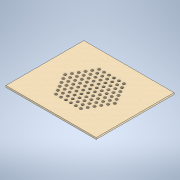
# Autodesk Inventor part: topPlatte
Saved by Autodesk Inventor 2020 (Build 240168000, 168)
## iProperties
Created: 2022-03-26
Part Number: topPlatte
Material: Pappel
Document SubType Name: Modeling
Designer: Eric
Density: 0.448 g/cm^3
Appearance: Pappel
Author: Eric
Autodesk Inventor part; units mm, degrees
ref_plane "YZ Plane" through (0, 0, 0) normal (1, 0, 0) x (0, 1, 0)
ref_plane "XZ Plane" through (0, 0, 0) normal (0, 1, 0) x (-1, 0, 0)
ref_plane "XY Plane" through (0, 0, 0) normal (0, 0, 1) x (1, 0, 0)
sketch "Skizze1" plane through (0, 0, 0) normal (0, 1, 0) x (-1, 0, 0)
  line L0 (0, 0) -> (-218, 0)
  line L1 (-218, 0) -> (-218, 188)
  line L2 (-218, 188) -> (0, 188)
  line L3 (0, 188) -> (0, 0)
  dimension "d0" = 188
  dimension "d1" = 218
  constraints: 8 end point, 2 parallel, 1 horizontal, 1 perpendicular
  measures "d0" distance of L2.end L0.start
  measures "d1" distance of L0.start L0.end
extrude "Extrusion1" add sketch "Skizze1" along normal blind 4
sketch "Skizze2" plane through (0, 0, 0) normal (0, -1, 0) x (1, 0, 0)
  circle A0 centre (109, 94) radius 3
  line L0 (103, 104.3923) -> (115, 104.3923) construction
  line L1 (115, 104.3923) -> (121, 94) construction
  line L2 (121, 94) -> (115, 83.6077) construction
  line L3 (115, 83.6077) -> (103, 83.6077) construction
  line L4 (103, 83.6077) -> (97, 94) construction
  line L5 (97, 94) -> (103, 104.3923) construction
  line L6 (97, 114.7846) -> (121, 114.7846) construction
  line L7 (121, 114.7846) -> (133, 94) construction
  line L8 (133, 94) -> (121, 73.2154) construction
  line L9 (121, 73.2154) -> (97, 73.2154) construction
  line L10 (97, 73.2154) -> (85, 94) construction
  line L11 (85, 94) -> (97, 114.7846) construction
  line L12 (85, 135.5692) -> (133, 135.5692) construction
  line L13 (157, 94) -> (133, 52.4308) construction
  line L14 (133, 52.4308) -> (85, 52.4308) construction
  line L15 (85, 52.4308) -> (61, 94) construction
  line L16 (61, 94) -> (85, 135.5692) construction
  line L17 (0, 0) -> (0, 188) projected
  line L18 (218, 0) -> (0, 0) construction
  line L19 (0, 0) -> (0, 188) projected
  line L20 (0, 94) -> (109, 94) construction
  line L21 (109, 94) -> (109, 0) construction
  line L22 (218, 0) -> (0, 0) construction
  circle A1 centre (103, 104.3923) radius 3
  circle A2 centre (115, 104.3923) radius 3
  circle A3 centre (121, 94) radius 3
  circle A4 centre (115, 83.6077) radius 3
  circle A5 centre (103, 83.6077) radius 3
  circle A6 centre (97, 94) radius 3
  circle A7 centre (85, 94) radius 3
  circle A8 centre (91, 104.3923) radius 3
  circle A9 centre (97, 114.7846) radius 3
  circle A10 centre (121, 114.7846) radius 3
  circle A11 centre (127, 104.3923) radius 3
  circle A12 centre (109, 114.7846) radius 3
  circle A13 centre (133, 94) radius 3
  circle A14 centre (127, 83.6077) radius 3
  circle A15 centre (121, 73.2154) radius 3
  circle A16 centre (109, 73.2154) radius 3
  circle A17 centre (97, 73.2154) radius 3
  circle A18 centre (91, 83.6077) radius 3
  circle A19 centre (85, 135.5692) radius 3
  circle A20 centre (73, 114.7846) radius 3
  circle A21 centre (79, 125.1769) radius 3
  circle A22 centre (67, 104.3923) radius 3
  circle A23 centre (61, 94) radius 3
  circle A24 centre (73, 73.2154) radius 3
  circle A25 centre (67, 83.6077) radius 3
  circle A26 centre (85, 52.4308) radius 3
  circle A27 centre (79, 62.8231) radius 3
  circle A28 centre (109, 52.4308) radius 3
  circle A29 centre (97, 52.4308) radius 3
  circle A30 centre (121, 52.4308) radius 3
  circle A31 centre (133, 52.4308) radius 3
  circle A32 centre (145, 73.2154) radius 3
  circle A33 centre (139, 62.8231) radius 3
  circle A34 centre (151, 83.6077) radius 3
  circle A35 centre (157, 94) radius 3
  circle A36 centre (145, 114.7846) radius 3
  circle A37 centre (151, 104.3923) radius 3
  circle A38 centre (139, 125.1769) radius 3
  circle A39 centre (133, 135.5692) radius 3
  circle A40 centre (109, 135.5692) radius 3
  circle A41 centre (121, 135.5692) radius 3
  circle A42 centre (97, 135.5692) radius 3
  line L23 (139, 125.1769) -> (133, 135.5692) construction
  line L24 (139, 125.1769) -> (145, 114.7846) construction
  line L25 (145, 114.7846) -> (151, 104.3923) construction
  line L26 (151, 104.3923) -> (157, 94) construction
  line L27 (151, 83.6077) -> (157, 94) construction
  line L28 (151, 83.6077) -> (145, 73.2154) construction
  line L29 (139, 62.8231) -> (145, 73.2154) construction
  line L30 (139, 62.8231) -> (133, 52.4308) construction
  line L31 (109, 52.4308) -> (121, 52.4308) construction
  line L32 (121, 52.4308) -> (133, 52.4308) construction
  line L33 (85, 52.4308) -> (97, 52.4308) construction
  line L34 (97, 52.4308) -> (109, 52.4308) construction
  line L35 (85, 52.4308) -> (79, 62.8231) construction
  line L36 (79, 62.8231) -> (73, 73.2154) construction
  line L37 (73, 73.2154) -> (67, 83.6077) construction
  line L38 (67, 83.6077) -> (61, 94) construction
  line L39 (61, 94) -> (67, 104.3923) construction
  line L40 (67, 104.3923) -> (73, 114.7846) construction
  line L41 (73, 114.7846) -> (79, 125.1769) construction
  line L42 (79, 125.1769) -> (85, 135.5692) construction
  line L43 (85, 135.5692) -> (97, 135.5692) construction
  line L44 (109, 135.5692) -> (97, 135.5692) construction
  line L45 (109, 135.5692) -> (121, 135.5692) construction
  line L46 (121, 135.5692) -> (133, 135.5692) construction
  line L47 (91, 125.1769) -> (103, 125.1769) construction
  line L48 (103, 125.1769) -> (115, 125.1769) construction
  line L49 (115, 125.1769) -> (127, 125.1769) construction
  line L50 (127, 125.1769) -> (133, 114.7846) construction
  line L51 (133, 114.7846) -> (139, 104.3923) construction
  line L52 (139, 104.3923) -> (145, 94) construction
  line L53 (145, 94) -> (139, 83.6077) construction
  line L54 (139, 83.6077) -> (133, 73.2154) construction
  line L55 (133, 73.2154) -> (127, 62.8231) construction
  line L56 (127, 62.8231) -> (115, 62.8231) construction
  line L57 (115, 62.8231) -> (103, 62.8231) construction
  line L58 (103, 62.8231) -> (91, 62.8231) construction
  line L59 (91, 62.8231) -> (85, 73.2154) construction
  line L60 (85, 73.2154) -> (79, 83.6077) construction
  line L61 (79, 83.6077) -> (73, 94) construction
  line L62 (73, 94) -> (79, 104.3923) construction
  line L63 (79, 104.3923) -> (85, 114.7846) construction
  line L64 (85, 114.7846) -> (91, 125.1769) construction
  line L65 (91, 125.1769) -> (127, 62.8231) construction
  circle A43 centre (73, 94) radius 3
  circle A44 centre (79, 104.3923) radius 3
  circle A45 centre (85, 114.7846) radius 3
  circle A46 centre (91, 125.1769) radius 3
  circle A47 centre (103, 125.1769) radius 3
  circle A48 centre (115, 125.1769) radius 3
  circle A49 centre (127, 125.1769) radius 3
  circle A50 centre (133, 114.7846) radius 3
  circle A51 centre (139, 104.3923) radius 3
  circle A52 centre (145, 94) radius 3
  circle A53 centre (139, 83.6077) radius 3
  circle A54 centre (133, 73.2154) radius 3
  circle A55 centre (127, 62.8231) radius 3
  circle A56 centre (115, 62.8231) radius 3
  circle A57 centre (103, 62.8231) radius 3
  circle A58 centre (91, 62.8231) radius 3
  circle A59 centre (85, 73.2154) radius 3
  circle A60 centre (79, 83.6077) radius 3
  line L66 (79, 145.9615) -> (91, 145.9615) construction
  line L67 (91, 145.9615) -> (103, 145.9615) construction
  line L68 (103, 145.9615) -> (115, 145.9615) construction
  line L69 (115, 145.9615) -> (127, 145.9615) construction
  line L70 (127, 145.9615) -> (139, 145.9615) construction
  line L71 (79, 145.9615) -> (73, 135.5692) construction
  line L72 (73, 135.5692) -> (67, 125.1769) construction
  line L73 (67, 125.1769) -> (61, 114.7846) construction
  line L74 (61, 114.7846) -> (55, 104.3923) construction
  line L75 (55, 104.3923) -> (49, 94) construction
  line L76 (139, 42.0385) -> (127, 42.0385) construction
  line L77 (127, 42.0385) -> (115, 42.0385) construction
  line L78 (115, 42.0385) -> (103, 42.0385) construction
  line L79 (103, 42.0385) -> (91, 42.0385) construction
  line L80 (91, 42.0385) -> (79, 42.0385) construction
  line L81 (169, 94) -> (163, 104.3923) construction
  line L82 (163, 104.3923) -> (157, 114.7846) construction
  line L83 (157, 114.7846) -> (151, 125.1769) construction
  line L84 (151, 125.1769) -> (145, 135.5692) construction
  line L85 (145, 135.5692) -> (139, 145.9615) construction
  line L86 (169, 94) -> (163, 83.6077) construction
  line L87 (163, 83.6077) -> (157, 73.2154) construction
  line L88 (157, 73.2154) -> (151, 62.8231) construction
  line L89 (151, 62.8231) -> (145, 52.4308) construction
  line L90 (145, 52.4308) -> (139, 42.0385) construction
  line L91 (79, 42.0385) -> (73, 52.4308) construction
  line L92 (73, 52.4308) -> (67, 62.8231) construction
  line L93 (67, 62.8231) -> (61, 73.2154) construction
  line L94 (61, 73.2154) -> (55, 83.6077) construction
  line L95 (55, 83.6077) -> (49, 94) construction
  line L96 (139, 42.0385) -> (79, 145.9615) construction
  circle A61 centre (49, 94) radius 3
  circle A62 centre (55, 104.3923) radius 3
  circle A63 centre (61, 114.7846) radius 3
  circle A64 centre (67, 125.1769) radius 3
  circle A65 centre (73, 135.5692) radius 3
  circle A66 centre (79, 145.9615) radius 3
  circle A67 centre (91, 145.9615) radius 3
  circle A68 centre (103, 145.9615) radius 3
  circle A69 centre (115, 145.9615) radius 3
  circle A70 centre (127, 145.9615) radius 3
  circle A71 centre (139, 145.9615) radius 3
  circle A72 centre (145, 135.5692) radius 3
  circle A73 centre (151, 125.1769) radius 3
  circle A74 centre (157, 114.7846) radius 3
  circle A75 centre (163, 104.3923) radius 3
  circle A76 centre (169, 94) radius 3
  circle A77 centre (163, 83.6077) radius 3
  circle A78 centre (157, 73.2154) radius 3
  circle A79 centre (151, 62.8231) radius 3
  circle A80 centre (145, 52.4308) radius 3
  circle A81 centre (139, 42.0385) radius 3
  circle A82 centre (79, 42.0385) radius 3
  circle A83 centre (91, 42.0385) radius 3
  circle A84 centre (103, 42.0385) radius 3
  circle A85 centre (115, 42.0385) radius 3
  circle A86 centre (127, 42.0385) radius 3
  circle A87 centre (73, 52.4308) radius 3
  circle A88 centre (67, 62.8231) radius 3
  circle A89 centre (61, 73.2154) radius 3
  circle A90 centre (55, 83.6077) radius 3
  dimension "d4" = 6
  dimension "d9" = 12
  dimension "d10" = 12
  dimension "d11" = 12
  dimension "d12" = 12
  dimension "d16" = 12
  constraints: 186 end point, 91 centre point, 90 equal radius, 69 coincident, 58 equal length, 48 point on line, 26 collinear, 15 midpoint, 8 horizontal, 2 horizontal alignment, 2 parallel, 2 perpendicular, 37 other
  measures "d4" diameter of A0
  measures "d9" distance of L0.end L1.end
  measures "d10" distance of L6.end A11.centre
  measures "d11" distance of L23.start L12.end
  measures "d12" distance of L49.end L50.end
  measures "d16" distance of L75.start L75.end
extrude "Extrusion2" cut sketch "Skizze2" against normal blind 4
equation "\"d10\" = d9"
equation "\"d11\" = d9"
equation "\"d12\" = d9"
equation "\"d16\" = d9"
